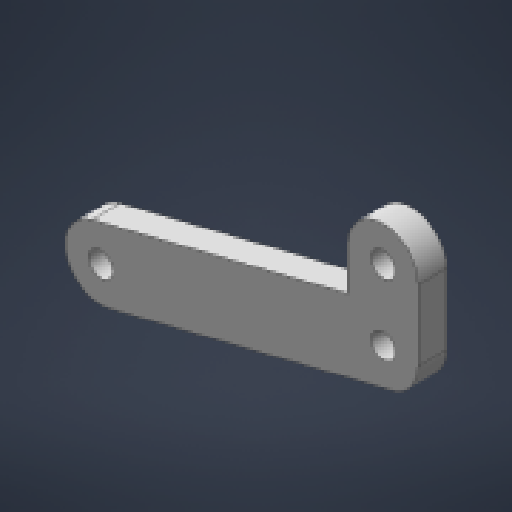
# Autodesk Inventor part: back_funnel
Saved by Autodesk Inventor 2025.2 (Build 292293000, 293)
## iProperties
Created: 2025-12-02
Part Number: back_funnel
Material: Generic
Document SubType Name: Modeling
Designer: cloudy
Density: 1 g/cm^3
Appearance: Smooth - Dark Gray
Author: cloudy
Autodesk Inventor part; units mm, degrees
ref_plane "YZ Plane" through (0, 0, 0) normal (1, 0, 0) x (0, 1, 0)
ref_plane "XZ Plane" through (0, 0, 0) normal (0, 1, 0) x (-1, 0, 0)
ref_plane "XY Plane" through (0, 0, 0) normal (0, 0, 1) x (1, 0, 0)
sketch "Sketch2" plane through (0, 0, 0) normal (0, 0, 1) x (1, 0, 0)
  circle A0 centre (-50.0249, -177.8) radius 2.1844
  circle A1 centre (0.7751, -165.1) radius 2.1844
  circle A2 centre (0.7751, -152.4) radius 2.1844
  circle A3 centre (-50.0249, -152.4) radius 2.1844
  circle A4 centre (0.7751, -165.1) radius 6.35
  circle A5 centre (0.7751, -152.4) radius 6.35
  circle A6 centre (-50.0249, -177.8) radius 6.35
  line L0 (-5.5749, -131.829) -> (-5.5749, -160.1421)
  line L1 (-5.5749, -160.1421) -> (-51.565, -171.6396)
  line L2 (-50.6267, -184.4959) -> (7.1251, -170.0579)
  line L3 (7.1251, -170.0579) -> (7.1251, -148.3402)
  line L4 (-35.2436, -141.802) -> (-32.4116, -141.802)
  line L5 (-29.119, -141.802) -> (-26.287, -141.802)
  spline S0 degree 2 poles (-32.1725, -141.802) (-30.7653, -141.3711) (-29.3581, -141.802) knots 0 0 0 1 1 1 weights 1 1.034831 1
  spline S1 degree 3 poles (-18.0653, -168.2172) (-18.4536, -168.2172) (-18.8762, -168.1704) (-19.697, -167.9732) (-20.0954, -167.8231) (-20.8527, -167.4498) (-21.2719, -167.1795) (-22.0369, -166.5475) (-22.3831, -166.1864) (-22.9733, -165.4543) (-23.2675, -165.0121) (-23.7675, -164.0794) (-23.9738, -163.5891) (-24.3066, -162.6061) (-24.4533, -162.017) (-24.6377, -160.8215) (-24.6757, -160.2153) (-24.6621, -159.1128) (-24.6099, -158.5123) (-24.3986, -157.3309) (-24.2392, -156.75) (-23.8884, -155.7901) (-23.676, -155.3161) (-23.1679, -154.4164) (-22.8717, -153.9909) (-22.2831, -153.29) (-21.9408, -152.9459) (-21.1885, -152.3448) (-20.778, -152.0883) (-20.039, -151.7346) (-19.651, -151.5925) (-18.8526, -151.4059) (-18.4422, -151.3617) (-17.7112, -151.3617) (-17.3252, -151.4007) (-16.572, -151.5661) (-16.2047, -151.6923) (-15.5081, -152.0046) (-15.1205, -152.2298) (-14.403, -152.7599) (-14.0727, -153.0644) (-13.4595, -153.7287) (-13.1325, -154.1611) (-12.571, -155.0834) (-12.3359, -155.573) (-11.9434, -156.5769) (-11.7643, -157.1906) (-11.5273, -158.4416) (-11.469, -159.0789) (-11.4545, -160.2496) (-11.4978, -160.8932) (-11.7067, -162.1597) (-11.8725, -162.7825) (-12.2466, -163.8115) (-12.4761, -164.3187) (-13.0308, -165.2763) (-13.3566, -165.7263) (-13.9735, -166.4214) (-14.3085, -166.7415) (-15.0395, -167.2999) (-15.436, -167.5376) (-16.1507, -167.8676) (-16.528, -168.0009) (-17.3028, -168.1759) (-17.7004, -168.2172) (-18.0653, -168.2172) knots 0 0 0 0 0.1165 0.1165 0.232999 0.232999 0.369785 0.369785 0.506571 0.506571 0.651905 0.651905 0.797238 0.797238 0.963262 0.963262 1.129286 1.129286 1.294016 1.294016 1.458745 1.458745 1.600629 1.600629 1.742513 1.742513 1.875203 1.875203 2.007893 2.007893 2.120972 2.120972 2.234051 2.234051 2.340282 2.340282 2.446513 2.446513 2.569309 2.569309 2.692105 2.692105 2.84053 2.84053 2.988954 2.988954 3.163874 3.163874 3.338794 3.338794 3.515132 3.515132 3.69147 3.69147 3.843605 3.843605 3.99574 3.99574 4.122409 4.122409 4.249078 4.249078 4.358558 4.358558 4.468037 4.468037 4.468037 4.468037
  ellipse E0 centre (-18.0653, -159.6619) end of major axis (-18.0653, -154.3017) minor radius 4
  ellipse E1 centre (-18.0653, -159.6619) end of major axis (-18.0653, -161.1359) minor radius 1.1
  ellipse E2 centre (-18.0653, -127.6068) end of major axis (-18.0653, -163.5416) minor radius 12.1199 (-21.7061, -161.8819) -> (-21.3672, -162.1823) ccw
  ellipse E3 centre (-18.0653, -159.6619) end of major axis (-18.0653, -154.3017) minor radius 4 (-22.0428, -160.2294) -> (-21.7061, -161.8819) ccw
  ellipse E4 centre (-18.0653, -180.8584) end of major axis (-18.0653, -204.6203) minor radius 8.0143 (-21.8601, -159.929) -> (-22.0428, -160.2294) ccw
  line L6 (-21.8601, -159.929) -> (-20.5574, -159.929)
  ellipse E5 centre (-18.0653, -159.6619) end of major axis (-18.0653, -163.012) minor radius 2.5 (-15.5733, -159.929) -> (-20.5574, -159.929) ccw
  line L7 (-15.5733, -159.929) -> (-14.2705, -159.929)
  ellipse E6 centre (-18.0653, -180.8584) end of major axis (-18.0653, -204.6203) minor radius 8.0143 (-14.0878, -160.2294) -> (-14.2705, -159.929) ccw
  ellipse E7 centre (-18.0653, -159.6619) end of major axis (-18.0653, -154.3017) minor radius 4 (-14.4245, -161.8819) -> (-14.0878, -160.2294) ccw
  ellipse E8 centre (-18.0653, -127.6068) end of major axis (-18.0653, -163.5416) minor radius 12.1199 (-14.7634, -162.1823) -> (-14.4245, -161.8819) ccw
  line L8 (-14.7634, -162.1823) -> (-16.4184, -162.1823)
  ellipse E9 centre (-18.0653, -159.6619) end of major axis (-18.0653, -163.012) minor radius 2.5 (-19.7122, -162.1823) -> (-16.4184, -162.1823) ccw
  line L9 (-19.7122, -162.1823) -> (-21.3672, -162.1823)
  ellipse E10 centre (-18.0653, -159.6619) end of major axis (-18.0653, -158.3218) minor radius 1
  line L10 (-41.3127, -175.622) -> (-8.3483, -167.3809)
  line L11 (-8.3483, -167.3809) -> (-5.5749, -160.1421)
  line L12 (-41.3127, -175.622) -> (-49.0132, -171.0017)
  point P0 (0, 0)
  point P1 (-48.4848, -183.9604)
  point P2 (2.3152, -171.2604)
  point P3 (7.1251, -165.1)
  point P4 (7.1251, -152.4)
  point P5 (-5.5749, -152.4)
  dimension "d6" = 12.7
  dimension "d9" = 135
  dimension "d10" = 125
  constraints: 26 end point, 6 horizontal, 6 tangent, 3 centre point, 3 coincident, 2 point on line, 1 equal radius, 1 horizontal alignment, 1 parallel, 77 other
  measures "d6" diameter of A5
  measures "d9" angle of L10 L12
  measures "d10" angle of L10 L11
extrude "Extrusion2" add sketch "Sketch2" along normal blind 5.08 contours A4 | A4 A5 L3 | A4 L2 A6 L12 L10 L11 L0 A5 | A5 | A6 | L1 L12 A6
fillet "Fillet1" radius 7.62 4 edges at (-49.0132, -171.0017, 2.54) (-41.3127, -175.622, 2.54) (-8.3483, -167.3809, 2.54) (-5.5749, -160.1421, 2.54)
body "Solid2"
